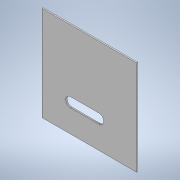
# Autodesk Inventor part: DecupajOvalizat
Saved by Autodesk Inventor 2022 (Build 260153000, 153)
## iProperties
Created: 2022-03-20
Part Number: DecupajOvalizat
Material: Generic
Document SubType Name: Sheet Metal
Designer: Janina
Density: 1 g/cm^3
Sheet Metal Rule: Default_mm
Appearance: Default
Author: Janina
Autodesk Inventor part; units mm, degrees
ref_plane "YZ Plane" through (0, 0, 0) normal (1, 0, 0) x (0, 1, 0)
ref_plane "XZ Plane" through (0, 0, 0) normal (0, 1, 0) x (-1, 0, 0)
ref_plane "XY Plane" through (0, 0, 0) normal (0, 0, 1) x (1, 0, 0)
sketch "Sketch1" plane through (0, 0, 0) normal (0, 0, 1) x (1, 0, 0)
  line L0 (-18.0403, 28.2997) -> (21.9597, 28.2997)
  line L1 (21.9597, 28.2997) -> (21.9597, -11.7003)
  line L2 (21.9597, -11.7003) -> (-18.0403, -11.7003)
  line L3 (-18.0403, -11.7003) -> (-18.0403, 28.2997)
  point P0 (0, 0)
  dimension "d0" = 40
  dimension "d1" = 40
  measures "d0" distance of L1.end L2.end
  measures "d1" distance of L0.end L1.end
extrude "Plate1" add sketch "Sketch1" along normal blind 0.5
sketch "Sketch2" plane through (0, 0, 0.5) normal (0, 0, 1) x (1, 0, 0)
  line L0 (6, 0) -> (-6, 0) construction
  line L1 (6, -2) -> (-6, -2)
  line L2 (-6, 2) -> (6, 2)
  arc A0 (6, -2) -> (6, 2) centre (6, 0) ccw
  arc A1 (-6, 2) -> (-6, -2) centre (-6, 0) ccw
  point P0 (0, 0)
  point P1 (0, 0)
  dimension "LG_C" = 12
  dimension "LT_C" = 4
  constraints: 8 end point, 4 point on circle, 4 tangent, 2 centre point, 1 coincident, 1 horizontal, 1 midpoint, 1 parallel
  measures "LG_C" distance of L0.start L0.end
  measures "LT_C" distance of L1.start L2.end
extrude "Cut1" cut sketch "Sketch2" against normal blind 0.5
equation "\"d6\" = Thickness"
equation "\"d2\" = Thickness"
equation "\"BendRadius\" = Thickness"
equation "\"BendReliefWidth\" = Thickness"
equation "\"BendReliefDepth\" = 0.5 * Thickness"
equation "\"CornerReliefSize\" = 4 * Thickness"
equation "\"MinimumRemnant\" = 2 * Thickness"
equation "\"TransitionRadius\" = BendRadius"
equation "\"JacobiRadiusSize\" = BendRadius"
equation "\"GapSize\" = Thickness"
equation "\"Thickness\" = 0.5"
body "Solid1"
